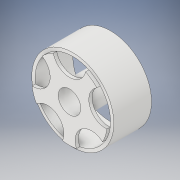
# Autodesk Inventor part: wheelMB
Saved by Autodesk Inventor 2017 (Build 210142000, 142)
## iProperties
Created: 2020-02-14
Part Number: wheelMB
Material: Generic
Document SubType Name: Modeling
Designer: 10023429
Density: 1 g/cm^3
Appearance: White
Author: 10023429
Autodesk Inventor part; units mm, degrees
ref_plane "YZ Plane" through (0, 0, 0) normal (1, 0, 0) x (0, 1, 0)
ref_plane "XZ Plane" through (0, 0, 0) normal (0, 1, 0) x (-1, 0, 0)
ref_plane "XY Plane" through (0, 0, 0) normal (0, 0, 1) x (1, 0, 0)
sketch "Sketch1" plane through (0, 0, 0) normal (0, 0, 1) x (1, 0, 0)
  circle A0 centre (0, 0) radius 5.588
  circle A1 centre (0, 0) radius 4.318
  circle A2 centre (0, 0) radius 14.478
  circle A3 centre (0, 0) radius 15.748
  dimension "d0" = 11.176
  dimension "d1" = 1.27
  dimension "d2" = 8.89
  dimension "d3" = 1.27
  constraints: 4 centre point, 1 coincident
  measures "d0" diameter of A0
  measures "d1" radial gap between concentric circles of A0 A1
  measures "d2" radial gap between concentric circles of A0 A2
  measures "d3" radial gap between concentric circles of A2 A3
extrude "Extrusion1" add sketch "Sketch1" along normal blind 14.478
sketch "Sketch2" plane through (0, 0, 14.478) normal (0, 0, 1) x (1, 0, 0)
  circle A0 centre (0, 0) radius 14.478 projected
  circle A1 centre (0, 0) radius 15.748 projected
  circle A2 centre (0, 0) radius 5.588 projected
  circle A3 centre (0, 0) radius 4.318 projected
  circle A4 centre (0, 0) radius 5.588 projected
extrude "Extrusion2" add sketch "Sketch2" along normal blind 1.27 contours A0 | A2
sketch "Sketch4" plane through (0, 0, 15.748) normal (0, 0, 1) x (1, 0, 0)
  circle A0 centre (0, 0) radius 14.478 projected
  circle A1 centre (0, 0) radius 4.318 projected
  circle A2 centre (0, 0) radius 14.478 projected
  arc A3 (-6.2014, 13.0826) -> (6.1895, 13.0883) centre (-0.0066, 14.478) ccw
  arc A4 (-14.3587, -1.8551) -> (-10.535, 9.931) centre (-13.7714, 4.4677) ccw
  arc A5 (-2.6728, -14.2292) -> (-12.7005, -6.9505) centre (-8.5046, -11.7168) ccw
  arc A6 (12.7068, -6.939) -> (2.6857, -14.2267) centre (8.5153, -11.7091) ccw
  arc A7 (10.526, 9.9406) -> (14.3603, -1.842) centre (13.7674, 4.4802) ccw
  dimension "d15" = 28.956
  dimension "d8" = 12.7
  dimension "d11" = 360
  dimension "d13" = 6.35
  dimension "d14" = 6.35
  dimension "d16" = 3.81
  dimension "d17" = 8.636
  constraints: 13 point on circle, 5 centre point, 23 other
  measures "d8" diameter of A3
  measures "d13" radius of A7
  measures "d14" radius of A3
  measures "d17" diameter of A1
extrude "Extrusion3" cut sketch "Sketch4" against normal blind 1.27 contours A3 A0
pattern_circular "Circular Pattern1" count 5 over 360 about axis through (0, 0, 14.478) along (0, 0, 1) of "Extrusion3"
body "Solid1"
